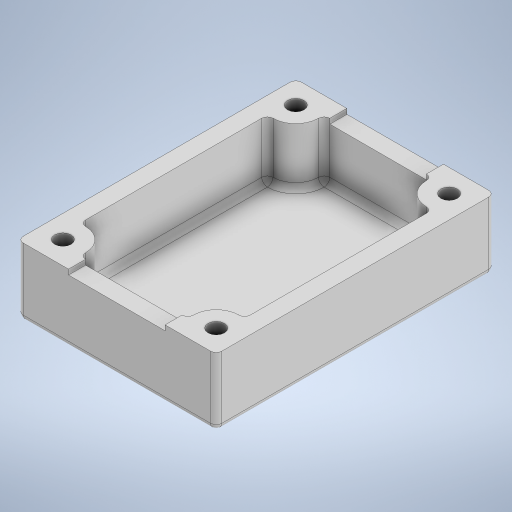
# Autodesk Inventor part: lid_V1
Saved by Autodesk Inventor 2023 (Build 270158000, 158)
## iProperties
Created: 2023-11-27
Part Number: lid_V1
Material: Generisch
Document SubType Name: Modeling
Designer: Mathi
Density: 1 g/cm^3
Appearance: Vorgabe
Author: Mathi
Autodesk Inventor part; units mm, degrees
ref_plane "YZ Plane" through (0, 0, 0) normal (1, 0, 0) x (0, 1, 0)
ref_plane "XZ Plane" through (0, 0, 0) normal (0, 1, 0) x (-1, 0, 0)
ref_plane "XY Plane" through (0, 0, 0) normal (0, 0, 1) x (1, 0, 0)
sketch "Skizze1" plane through (0, 0, 0) normal (0, 1, 0) x (-1, 0, 0)
  line L0 (-17.5, 24.5) -> (17.5, 24.5)
  line L1 (17.5, 24.5) -> (17.5, -24.5)
  line L2 (17.5, -24.5) -> (-17.5, -24.5)
  line L3 (-17.5, -24.5) -> (-17.5, 24.5)
  line L4 (-17.5, 24.5) -> (17.5, -24.5) construction
  line L5 (17.5, 24.5) -> (-17.5, -24.5) construction
  line L6 (14.5, -21.5) -> (14.5, 21.5)
  line L7 (14.5, 21.5) -> (-14.5, 21.5)
  line L8 (-14.5, 21.5) -> (-14.5, -21.5)
  line L9 (-14.5, -21.5) -> (14.5, -21.5)
  line L10 (8.5, 24.5) -> (8.5, 21.5)
  line L11 (-8.5, 24.5) -> (-8.5, 21.5)
  line L12 (-13.5, -20.5) -> (13.5, -20.5) construction
  line L13 (13.5, -20.5) -> (13.5, 20.5) construction
  line L14 (13.5, 20.5) -> (-13.5, 20.5) construction
  line L15 (-13.5, 20.5) -> (-13.5, -20.5) construction
  line L16 (-13.5, -20.5) -> (13.5, 20.5) construction
  line L17 (13.5, -20.5) -> (-13.5, 20.5) construction
  circle A0 centre (13.5, 20.5) radius 4
  circle A1 centre (13.5, -20.5) radius 4
  circle A2 centre (-13.5, -20.5) radius 4
  circle A3 centre (-13.5, 20.5) radius 4
  line L18 (8.5, -21.5) -> (8.5, -24.5)
  line L19 (-8.5, -21.5) -> (-8.5, -24.5)
  line L20 (-8.5, 23) -> (8.5, 23) construction
  line L21 (8.5, -23) -> (-8.5, -23) construction
  line L22 (0, 21.5) -> (0, 0) construction
  point P0 (14.5, -16.627)
  point P1 (9.627, -21.5)
  point P2 (-9.627, -21.5)
  point P3 (-14.5, -16.627)
  point P4 (-14.5, 16.627)
  point P5 (-9.627, 21.5)
  point P6 (9.627, 21.5)
  point P7 (14.5, 16.627)
  dimension "d0" = 49
  dimension "d1" = 35
  dimension "d2" = 3
  dimension "d22" = 27
  dimension "d23" = 41
  dimension "d24" = 8
  dimension "d31" = 17
  constraints: 46 end point, 10 point on line, 9 midpoint, 7 parallel, 7 perpendicular, 4 centre point, 3 coincident, 3 equal radius, 2 horizontal, 1 vertical, 5 other
  measures "d0" distance of L0.end L1.end
  measures "d1" distance of L0.start L0.end
  measures "d2" distance between parallel lines of L8 L3
  measures "d22" distance of L14.end L13.end
  measures "d23" distance of L13.end L12.end
  measures "d24" diameter of A0
  measures "d31" diameter of L10 L22
extrude "Extrusion1" add sketch "Skizze1" along normal blind 10 contours L11 L7 A3 L0 | L0 L10 L7 L11 | L0 A0 L7 L10 | A3 L3 L0 | A3 L7 L8 | L0 L1 A0 | A0 L6 L7 | A3 L8 L7 | A3 L8 A2 L3 | L1 A1 L6 A0 | L7 L6 A0 | A2 L2 L3 | A2 L8 L9 | A1 L9 L6 | L1 L2 A1 | A2 L9 L8 | A2 L9 L19 L2 | L6 L9 A1 | L2 L18 L9 A1 | L19 L9 L18 L2
extrude "Extrusion2" add sketch "Skizze1" against normal blind 2
sketch "Skizze2" plane through (0, 10, 0) normal (0, 1, 0) x (1, 0, 0)
  line L0 (8.5, -24.5) -> (8.5, -21.5) projected
  line L1 (-8.5, -24.5) -> (-8.5, -21.5) projected
  line L2 (-8.5, -24.5) -> (8.5, -24.5)
  line L3 (-17.5, -24.5) -> (17.5, -24.5) projected
  line L4 (-8.5, -21.5) -> (8.5, -21.5)
  line L5 (9.627, -21.5) -> (-9.627, -21.5) projected
  line L6 (-8.5, 21.5) -> (-8.5, 24.5) projected
  line L7 (8.5, 21.5) -> (8.5, 24.5) projected
  line L8 (-8.5, 21.5) -> (8.5, 21.5)
  line L9 (-9.627, 21.5) -> (9.627, 21.5) projected
  line L10 (-8.5, 24.5) -> (8.5, 24.5)
  line L11 (17.5, 24.5) -> (-17.5, 24.5) projected
  point P0 (0, 0)
  point P1 (-2.5, -21.5)
  point P2 (-12.5, -19.5)
  point P3 (-9.627, -21.5)
  constraints: 8 end point, 3 collinear, 1 horizontal, 1 other
extrude "Extrusion3" cut sketch "Skizze2" against normal blind 0.9
fillet "Rundung1" radius 1 23 edges at (-17.5, 4, -24.5) (-17.5, 4, 24.5) (14.5, 0, 0) (0, 0, 21.5) (-14.5, 0, 0) (0, 0, -21.5) (0, -2, -24.5) (-17.5, -2, 0) (17.5, -2, 0) (0, -2, 24.5) (-14.5, 5, -16.627) (-9.627, 5, -21.5) (9.627, 5, -21.5) (14.5, 5, -16.627) (10.6716, 0, -17.6716) (-10.6716, 0, -17.6716) (10.6716, 0, 17.6716) (14.5, 5, 16.627) (9.627, 5, 21.5) (-9.627, 5, 21.5) (-14.5, 5, 16.627) (17.5, 4, -24.5) (17.5, 4, 24.5)
sketch "Skizze3" plane through (0, -2, 0) normal (0, -1, 0) x (1, 0, 0)
  point P0 (13.5, -20.5)
  point P1 (13.5, 20.5)
  point P2 (-13.5, 20.5)
  point P3 (-13.5, 20.5)
  point P4 (-13.5, -20.5)
  point P5 (13.5, -20.5)
  point P6 (13.5, 20.5)
  point P7 (-13.5, -20.5)
  constraints: 4 coincident
hole "Bohrung1" at (13.5, -2, -20.5) at (13.5, -2, 20.5) at (-13.5, -2, 20.5) at (-13.5, -2, -20.5) direction (0, 1, 0) diameter 2.9 end through all counterbore diameter 5.5 counterbore depth 10 clearance for "Inbusschraube DIN EN ISO 4762" size "M2.5" standard "DIN"
sketch "Skizze4" plane through (0, -2, 0) normal (0, -1, 0) x (1, 0, 0)
  line L0 (3.25, 21.5) -> (3.25, -21.5) construction
  line L1 (3.25, -21.5) -> (-3.25, -21.5) construction
  line L2 (-3.25, -21.5) -> (-3.25, 21.5) construction
  line L3 (-3.25, 21.5) -> (3.25, 21.5) construction
  line L4 (-3.25, 21.5) -> (3.25, -21.5) construction
  spline S0 degree 2 poles (3.25, 18.2103) (3.25, 17.2845) (2.4887, 15.9357) (1.0929, 15.2496) (0.1624, 15.2496) knots 0 0 0 1 2 3 3 3
  spline S1 degree 2 poles (0.1624, 15.2496) (-0.5284, 15.2496) (-1.6657, 15.6256) (-2.5069, 16.3822) (-2.9487, 17.4819) (-2.9487, 18.1868) knots 0 0 0 1 2 3 4 4 4
  spline S2 degree 2 poles (-2.9487, 18.1868) (-2.9487, 18.8918) (-2.4928, 20.0055) (-1.661, 20.7528) (-0.5002, 21.1334) (0.1671, 21.1334) knots 0 0 0 1 2 3 4 4 4
  spline S3 degree 2 poles (0.1671, 21.1334) (0.8532, 21.1334) (2.0046, 20.7387) (2.8176, 19.982) (3.25, 18.8965) (3.25, 18.2103) knots 0 0 0 1 2 3 4 4 4
  spline S4 degree 2 poles (0.1671, 16.6172) (0.7921, 16.6172) (1.6898, 17.0119) (2.1456, 17.7404) (2.1456, 18.2103) knots 0 0 0 1 2 3 3 3
  spline S5 degree 2 poles (2.1456, 18.2103) (2.1456, 18.5487) (1.8918, 19.1126) (1.4125, 19.5215) (0.6465, 19.7659) (0.1671, 19.7659) knots 0 0 0 1 2 3 4 4 4
  spline S6 degree 2 poles (0.1671, 19.7659) (-0.3169, 19.7659) (-1.0971, 19.5215) (-1.5999, 19.0891) (-1.8443, 18.5346) (-1.8443, 18.1962) knots 0 0 0 1 2 3 4 4 4
  spline S7 degree 2 poles (-1.8443, 18.1962) (-1.8443, 17.7639) (-1.4166, 17.0495) (-0.5049, 16.6172) (0.1671, 16.6172) knots 0 0 0 1 2 3 3 3
  line L5 (-1.8067, 12.2983) -> (1.7461, 13.0643)
  line L6 (1.7461, 13.0643) -> (-2.1968, 13.0643)
  spline S8 degree 2 poles (-2.1968, 13.0643) (-2.5633, 13.0643) (-2.9487, 13.4121) (-2.9487, 13.6941) knots 0 0 0 1 2 2 2
  spline S9 degree 2 poles (-2.9487, 13.6941) (-2.9487, 13.9713) (-2.568, 14.3191) (-2.1968, 14.3191) knots 0 0 0 1 2 2 2
  line L7 (-2.1968, 14.3191) -> (2.4229, 14.3191)
  spline S10 degree 2 poles (2.4229, 14.3191) (2.8458, 14.3191) (3.1513, 13.8633) (3.1513, 13.4967) knots 0 0 0 1 2 2 2
  line L8 (3.1513, 13.4967) -> (3.1513, 13.1348)
  spline S11 degree 2 poles (3.1513, 13.1348) (3.1513, 12.7871) (3.0103, 12.4393) (2.672, 12.2842) (2.3101, 12.1902) knots 0 0 0 1 2 3 3 3
  line L9 (2.3101, 12.1902) -> (-0.8198, 11.4242)
  line L10 (-0.8198, 11.4242) -> (2.3101, 10.6582)
  spline S12 degree 2 poles (2.3101, 10.6582) (2.672, 10.5642) (3.0103, 10.4044) (3.1513, 10.0566) (3.1513, 9.7089) knots 0 0 0 1 2 3 3 3
  line L11 (3.1513, 9.7089) -> (3.1513, 9.347)
  spline S13 degree 2 poles (3.1513, 9.347) (3.1513, 8.9804) (2.8458, 8.5246) (2.4229, 8.5246) knots 0 0 0 1 2 2 2
  line L12 (2.4229, 8.5246) -> (-2.1968, 8.5246)
  spline S14 degree 2 poles (-2.1968, 8.5246) (-2.5633, 8.5246) (-2.9487, 8.8723) (-2.9487, 9.159) knots 0 0 0 1 2 2 2
  spline S15 degree 2 poles (-2.9487, 9.159) (-2.9487, 9.4316) (-2.5633, 9.7794) (-2.1968, 9.7794) knots 0 0 0 1 2 2 2
  line L13 (-2.1968, 9.7794) -> (1.7461, 9.7794)
  line L14 (1.7461, 9.7794) -> (-1.9054, 10.5501)
  spline S16 degree 2 poles (-1.9054, 10.5501) (-2.2626, 10.6394) (-2.6338, 10.7663) (-2.9487, 11.114) (-2.9487, 11.4195) knots 0 0 0 1 2 3 3 3
  spline S17 degree 2 poles (-2.9487, 11.4195) (-2.9487, 11.6545) (-2.7466, 11.9787) (-2.4411, 12.1526) (-2.0887, 12.2466) (-1.8067, 12.2983) knots 0 0 0 1 2 3 4 4 4
  spline S18 degree 2 poles (-1.0125, 2.7347) (-1.567, 2.7347) (-2.4552, 3.3081) (-2.9487, 4.3937) (-2.9487, 5.1362) knots 0 0 0 1 2 3 3 3
  spline S19 degree 2 poles (-2.9487, 5.1362) (-2.9487, 6.0244) (-2.615, 6.6025) knots 0 0 0 1 1 1
  spline S20 degree 2 poles (-2.615, 6.6025) (-2.3659, 7.0207) (-1.5482, 7.5424) (-1.1488, 7.5424) knots 0 0 0 1 2 2 2
  spline S21 degree 2 poles (-1.1488, 7.5424) (-0.9044, 7.5424) (-0.5472, 7.1946) (-0.5472, 6.9267) knots 0 0 0 1 2 2 2
  spline S22 degree 2 poles (-0.5472, 6.9267) (-0.5472, 6.7059) (-0.8245, 6.4098) (-1.0736, 6.3111) knots 0 0 0 1 2 2 2
  spline S23 degree 2 poles (-1.0736, 6.3111) (-1.3461, 6.203) (-1.6986, 5.9586) (-1.9195, 5.531) (-1.9195, 5.1691) knots 0 0 0 1 2 3 3 3
  spline S24 degree 2 poles (-1.9195, 5.1691) (-1.9195, 4.671) (-1.4683, 4.0694) (-1.1441, 4.0694) knots 0 0 0 1 2 2 2
  spline S25 degree 2 poles (-1.1441, 4.0694) (-0.8856, 4.0694) (-0.5613, 4.3843) (-0.3827, 4.92) (-0.2747, 5.39) knots 0 0 0 1 2 3 3 3
  spline S26 degree 2 poles (-0.2747, 5.39) (-0.1243, 6.0291) (0.2846, 6.9032) (1.0036, 7.4296) (1.5394, 7.4296) knots 0 0 0 1 2 3 3 3
  spline S27 degree 2 poles (1.5394, 7.4296) (2.0422, 7.4296) (2.8317, 6.875) (3.25, 5.8411) (3.25, 5.1503) knots 0 0 0 1 2 3 3 3
  spline S28 degree 2 poles (3.25, 5.1503) (3.25, 4.6005) (2.9727, 3.7874) (2.5075, 3.2423) (1.9952, 2.9885) (1.7461, 2.9885) knots 0 0 0 1 2 3 4 4 4
  spline S29 degree 2 poles (1.7461, 2.9885) (1.5065, 2.9885) (1.1117, 3.3363) (1.1117, 3.5948) knots 0 0 0 1 2 2 2
  spline S30 degree 2 poles (1.1117, 3.5948) (1.1117, 3.8344) (1.3467, 4.0788) (1.577, 4.201) knots 0 0 0 1 2 2 2
  spline S31 degree 2 poles (1.577, 4.201) (1.9059, 4.3608) (2.249, 4.7696) (2.249, 5.2302) knots 0 0 0 1 2 2 2
  spline S32 degree 2 poles (2.249, 5.2302) (2.249, 5.6579) (1.8871, 6.1654) (1.6475, 6.1654) knots 0 0 0 1 2 2 2
  spline S33 degree 2 poles (1.6475, 6.1654) (1.4971, 6.1654) (1.2762, 6.0009) (1.107, 5.6908) (1.0083, 5.3618) (0.9049, 4.9482) knots 0 0 0 1 2 3 4 4 4
  spline S34 degree 2 poles (0.9049, 4.9482) (0.7921, 4.4689) (0.5055, 3.6512) (0.0919, 3.0684) (-0.5566, 2.7347) (-1.0125, 2.7347) knots 0 0 0 1 2 3 4 4 4
  line L15 (0.9378, 0.6059) -> (-2.2015, 0.6059)
  spline S35 degree 2 poles (-2.2015, 0.6059) (-2.5633, 0.6059) (-2.9487, 0.963) (-2.9487, 1.2403) knots 0 0 0 1 2 2 2
  spline S36 degree 2 poles (-2.9487, 1.2403) (-2.9487, 1.5176) (-2.5539, 1.8606) (-2.2015, 1.8606) knots 0 0 0 1 2 2 2
  line L16 (-2.2015, 1.8606) -> (0.9049, 1.8606)
  spline S37 degree 2 poles (0.9049, 1.8606) (1.2574, 1.8606) (1.6334, 1.5176) (1.6334, 1.2403) knots 0 0 0 1 2 2 2
  spline S38 degree 2 poles (1.6334, 1.2403) (1.6334, 0.963) (1.2574, 0.6059) (0.9378, 0.6059) knots 0 0 0 1 2 2 2
  spline S39 degree 2 poles (1.9764, 1.2262) (1.9764, 1.4847) (2.3007, 1.8606) (2.5921, 1.8606) knots 0 0 0 1 2 2 2
  spline S40 degree 2 poles (2.5921, 1.8606) (2.8599, 1.8606) (3.203, 1.48) (3.203, 1.2262) knots 0 0 0 1 2 2 2
  spline S41 degree 2 poles (3.203, 1.2262) (3.203, 0.9865) (2.8881, 0.6059) (2.5921, 0.6059) knots 0 0 0 1 2 2 2
  spline S42 degree 2 poles (2.5921, 0.6059) (2.3054, 0.6059) (1.9764, 0.9771) (1.9764, 1.2262) knots 0 0 0 1 2 2 2
  spline S43 degree 2 poles (-2.9487, -1.2035) (-2.9487, -0.9215) (-2.5821, -0.5126) (-2.2579, -0.5126) knots 0 0 0 1 2 2 2
  spline S44 degree 2 poles (-2.2579, -0.5126) (-1.9853, -0.5126) (-1.5858, -0.9027) (-1.5858, -1.1894) knots 0 0 0 1 2 2 2
  spline S45 degree 2 poles (-1.5858, -1.1894) (-1.5858, -1.476) (-1.9806, -1.8802) (-2.2579, -1.8802) knots 0 0 0 1 2 2 2
  spline S46 degree 2 poles (-2.2579, -1.8802) (-2.5774, -1.8802) (-2.9487, -1.476) (-2.9487, -1.2035) knots 0 0 0 1 2 2 2
  line L17 (-2.85, -5.6586) -> (-2.85, -3.8775)
  spline S47 degree 2 poles (-2.85, -3.8775) (-2.85, -3.4498) (-2.4552, -3.0739) (-2.0417, -3.0739) knots 0 0 0 1 2 2 2
  line L18 (-2.0417, -3.0739) -> (2.3477, -3.0739)
  spline S48 degree 2 poles (2.3477, -3.0739) (2.7659, -3.0739) (3.1513, -3.4592) (3.1513, -3.8775) knots 0 0 0 1 2 2 2
  line L19 (3.1513, -3.8775) -> (3.1513, -5.7667)
  spline S49 degree 2 poles (3.1513, -5.7667) (3.1513, -6.1897) (3.0432, -6.8288) (2.8411, -7.1249) knots 0 0 0 1 2 2 2
  spline S50 degree 2 poles (2.8411, -7.1249) (2.7565, -7.3035) (2.3571, -7.6418) (1.873, -7.8204) (1.6052, -7.8204) knots 0 0 0 1 2 3 3 3
  spline S51 degree 2 poles (1.6052, -7.8204) (0.6747, -7.8204) (0.3363, -6.9416) knots 0 0 0 1 1 1
  spline S52 degree 2 poles (0.3363, -6.9416) (0.0167, -8.093) (-1.1018, -8.093) knots 0 0 0 1 1 1
  spline S53 degree 2 poles (-1.1018, -8.093) (-1.614, -8.093) (-2.4411, -7.5619) (-2.6479, -7.0779) knots 0 0 0 1 2 2 2
  spline S54 degree 2 poles (-2.6479, -7.0779) (-2.756, -6.8382) (-2.85, -6.1333) (-2.85, -5.6586) knots 0 0 0 1 2 2 2
  line L20 (-0.2559, -5.5693) -> (-0.2559, -4.4227)
  line L21 (-0.2559, -4.4227) -> (-1.7973, -4.4227)
  line L22 (-1.7973, -4.4227) -> (-1.7973, -5.6116)
  spline S55 degree 2 poles (-1.7973, -5.6116) (-1.7973, -6.7254) (-1.0125, -6.7254) knots 0 0 0 1 1 1
  spline S56 degree 2 poles (-1.0125, -6.7254) (-0.6177, -6.7254) (-0.2559, -6.1615) (-0.2559, -5.5693) knots 0 0 0 1 2 2 2
  line L23 (2.0986, -4.4227) -> (0.7545, -4.4227)
  line L24 (0.7545, -4.4227) -> (0.7545, -5.4237)
  spline S57 degree 2 poles (0.7545, -5.4237) (0.7545, -5.8513) (0.9049, -6.2884) (1.0929, -6.3918) knots 0 0 0 1 2 2 2
  spline S58 degree 2 poles (1.0929, -6.3918) (1.2621, -6.4904) (1.4501, -6.4904) knots 0 0 0 1 1 1
  spline S59 degree 2 poles (1.4501, -6.4904) (1.8354, -6.4904) (2.0986, -5.9218) (2.0986, -5.2968) knots 0 0 0 1 2 2 2
  line L25 (2.0986, -5.2968) -> (2.0986, -4.4227)
  line L26 (0.9378, -10.2501) -> (-2.2015, -10.2501)
  spline S60 degree 2 poles (-2.2015, -10.2501) (-2.5633, -10.2501) (-2.9487, -9.8929) (-2.9487, -9.6156) knots 0 0 0 1 2 2 2
  spline S61 degree 2 poles (-2.9487, -9.6156) (-2.9487, -9.3384) (-2.5539, -8.9953) (-2.2015, -8.9953) knots 0 0 0 1 2 2 2
  line L27 (-2.2015, -8.9953) -> (0.9049, -8.9953)
  spline S62 degree 2 poles (0.9049, -8.9953) (1.2574, -8.9953) (1.6334, -9.3384) (1.6334, -9.6156) knots 0 0 0 1 2 2 2
  spline S63 degree 2 poles (1.6334, -9.6156) (1.6334, -9.8929) (1.2574, -10.2501) (0.9378, -10.2501) knots 0 0 0 1 2 2 2
  spline S64 degree 2 poles (1.9764, -9.6297) (1.9764, -9.3713) (2.3007, -8.9953) (2.5921, -8.9953) knots 0 0 0 1 2 2 2
  spline S65 degree 2 poles (2.5921, -8.9953) (2.8599, -8.9953) (3.203, -9.376) (3.203, -9.6297) knots 0 0 0 1 2 2 2
  spline S66 degree 2 poles (3.203, -9.6297) (3.203, -9.8694) (2.8881, -10.2501) (2.5921, -10.2501) knots 0 0 0 1 2 2 2
  spline S67 degree 2 poles (2.5921, -10.2501) (2.3054, -10.2501) (1.9764, -9.8788) (1.9764, -9.6297) knots 0 0 0 1 2 2 2
  line L28 (-2.3988, -13.9674) -> (-0.8762, -13.0651)
  line L29 (-0.8762, -13.0651) -> (-1.3837, -12.581)
  line L30 (-1.3837, -12.581) -> (-2.2109, -12.581)
  spline S68 degree 2 poles (-2.2109, -12.581) (-2.5586, -12.581) (-2.9487, -12.2004) (-2.9487, -11.9513) knots 0 0 0 1 2 2 2
  spline S69 degree 2 poles (-2.9487, -11.9513) (-2.9487, -11.6599) (-2.5633, -11.331) (-2.2015, -11.331) knots 0 0 0 1 2 2 2
  line L31 (-2.2015, -11.331) -> (2.4276, -11.331)
  spline S70 degree 2 poles (2.4276, -11.331) (2.8176, -11.331) (3.25, -11.6505) (3.25, -11.9513) knots 0 0 0 1 2 2 2
  spline S71 degree 2 poles (3.25, -11.9513) (3.25, -12.2427) (2.8552, -12.581) (2.4934, -12.581) knots 0 0 0 1 2 2 2
  line L32 (2.4934, -12.581) -> (-0.0585, -12.581)
  line L33 (-0.0585, -12.581) -> (1.1963, -13.6572)
  spline S72 degree 2 poles (1.1963, -13.6572) (1.4313, -13.8828) (1.6334, -14.1554) (1.6334, -14.3575) knots 0 0 0 1 2 2 2
  spline S73 degree 2 poles (1.6334, -14.3575) (1.6334, -14.5925) (1.3279, -14.912) (1.0976, -14.912) knots 0 0 0 1 2 2 2
  spline S74 degree 2 poles (1.0976, -14.912) (0.825, -14.912) (0.4632, -14.4703) knots 0 0 0 1 1 1
  line L34 (0.4632, -14.4703) -> (-0.082, -13.8969)
  line L35 (-0.082, -13.8969) -> (-1.7738, -14.9966)
  spline S75 degree 2 poles (-1.7738, -14.9966) (-1.9618, -15.1141) (-2.2015, -15.241) (-2.3049, -15.241) knots 0 0 0 1 2 2 2
  spline S76 degree 2 poles (-2.3049, -15.241) (-2.6009, -15.241) (-2.9487, -14.912) (-2.9487, -14.6441) knots 0 0 0 1 2 2 2
  spline S77 degree 2 poles (-2.9487, -14.6441) (-2.9487, -14.4045) (-2.709, -14.1648) (-2.3988, -13.9674) knots 0 0 0 1 2 2 2
  line L36 (-1.0078, -19.1369) -> (-1.0078, -17.0973)
  spline S78 degree 2 poles (-1.0078, -17.0973) (-1.2757, -17.102) (-1.802, -17.3699) (-2.0652, -17.8116) (-2.0652, -18.0795) knots 0 0 0 1 2 3 3 3
  spline S79 degree 2 poles (-2.0652, -18.0795) (-2.0652, -18.2628) (-1.9806, -18.5589) (-1.802, -18.8408) (-1.5576, -19.1181) (-1.3837, -19.3014) knots 0 0 0 1 2 3 4 4 4
  spline S80 degree 2 poles (-1.3837, -19.3014) (-1.2945, -19.4095) (-1.2945, -19.5975) knots 0 0 0 1 1 1
  spline S81 degree 2 poles (-1.2945, -19.5975) (-1.2945, -19.7948) (-1.5247, -20.0533) (-1.7221, -20.0533) knots 0 0 0 1 2 2 2
  spline S82 degree 2 poles (-1.7221, -20.0533) (-1.8913, -20.0533) (-2.319, -19.8042) (-2.6996, -19.3155) (-2.9487, -18.5824) (-2.9487, -18.1124) knots 0 0 0 1 2 3 4 4 4
  spline S83 degree 2 poles (-2.9487, -18.1124) (-2.9487, -17.0268) (-1.7033, -15.819) (-0.6459, -15.819) knots 0 0 0 1 2 2 2
  spline S84 degree 2 poles (-0.6459, -15.819) (-0.1478, -15.819) (0.6982, -16.1151) (1.3138, -16.6884) (1.6428, -17.525) (1.6428, -18.0325) knots 0 0 0 1 2 3 4 4 4
  spline S85 degree 2 poles (1.6428, -18.0325) (1.6428, -18.6904) (1.0788, -19.6445) (0.1906, -20.1191) (-0.27, -20.1191) knots 0 0 0 1 2 3 3 3
  spline S86 degree 2 poles (-0.27, -20.1191) (-0.7305, -20.1191) (-1.0078, -19.5834) (-1.0078, -19.1369) knots 0 0 0 1 2 2 2
  line L37 (-0.2277, -17.0973) -> (-0.2277, -18.8972)
  spline S87 degree 2 poles (-0.2277, -18.8972) (0.2141, -18.8596) (0.7216, -18.385) (0.7216, -17.9949) knots 0 0 0 1 2 2 2
  spline S88 degree 2 poles (0.7216, -17.9949) (0.7216, -17.6284) (0.2047, -17.149) (-0.2277, -17.0973) knots 0 0 0 1 2 2 2
  point P0 (0, 0)
  point P1 (0, 0)
  dimension "d26" = 43
  dimension "d27" = 6.5
  constraints: 2 end point, 1 coincident, 1 midpoint, 1 vertical, 2 other
  measures "d26" distance of L0.start L0.end
  measures "d27" distance of L2.end L0.start
extrude "Extrusion4" cut sketch "Skizze4" against normal blind 0.5
